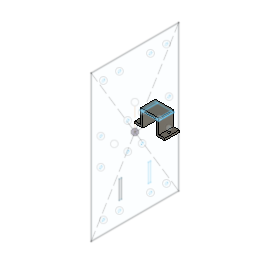
Chassis frame v6-2 (Autodesk Fusion 360 design; units mm, degrees)
Autodesk Fusion 360 part; units mm, degrees
sketch "Sketch1" plane through (0, 0, 0) normal (1, 0, 0) x (0, 1, 0) in component "Integrated frame"
  circle A0 centre (-46.8244, 18.5) radius 1.5
  circle A1 centre (-9.8244, 18.5) radius 1.5
  circle A2 centre (-46.8244, -18.5) radius 1.5
  circle A3 centre (-9.8244, -18.5) radius 1.5
  line L0 (0, 0) -> (0, 35.4619) construction
  line L1 (60, 100) -> (-60, 100)
  line L2 (-60, 100) -> (-60, -100)
  line L3 (-60, -100) -> (60, -100)
  line L4 (60, -100) -> (60, 100)
  line L5 (60, 100) -> (-60, -100) construction
  line L6 (-60, 100) -> (60, -100) construction
  circle A4 centre (46.8244, 18.5) radius 1.5
  circle A5 centre (46.8244, -18.5) radius 1.5
  circle A6 centre (9.8244, -18.5) radius 1.5
  circle A7 centre (9.8244, 18.5) radius 1.5
  line L7 (-18.5, -45.3481) -> (-21.5, -45.3481)
  line L8 (-21.5, -45.3481) -> (-21.5, -70.3481)
  line L9 (-21.5, -70.3481) -> (-18.5, -70.3481)
  line L10 (-18.5, -70.3481) -> (-18.5, -45.3481)
  line L11 (21.5, -45.3481) -> (21.5, -70.3481)
  line L12 (18.5, -70.3481) -> (18.5, -45.3481)
  line L13 (18.5, -45.3481) -> (21.5, -45.3481)
  line L14 (21.5, -70.3481) -> (18.5, -70.3481)
  circle A8 centre (-43.3091, 82.7998) radius 1.5
  circle A9 centre (-21.3091, 82.7998) radius 1.5
  circle A10 centre (21.3091, 82.7998) radius 1.5
  circle A11 centre (43.3091, 82.7998) radius 1.5
  line L15 (0, 0) -> (33.4715, 0) construction
  circle A12 centre (-43.3091, -82.7998) radius 1.5
  circle A13 centre (-21.3091, -82.7998) radius 1.5
  circle A14 centre (43.3091, -82.7998) radius 1.5
  circle A15 centre (21.3091, -82.7998) radius 1.5
  point P0 (-28.3244, 0)
  dimension "d246" = 3
  dimension "d248" = 18.5
  dimension "d249" = 18.5
  dimension "d252" = 37
  dimension "d253" = -37
  dimension "d261" = 120
  dimension "d262" = 200
  dimension "d264" = 3
  dimension "d265" = 25
  dimension "d266" = 18.5
  dimension "d269" = 3
  dimension "d270" = 3
  dimension "d271" = 22
  constraint coincident L0.start L15.start
  constraint horizontal L1
  constraint perpendicular L1 L2
  constraint parallel L1 L3
  constraint parallel L2 L4
  constraint coincident L5 L0.start
  constraint coincident L6 L0.start
  constraint symmetric A0 L0 A4
  constraint symmetric A1 L0 A7
  constraint symmetric A2 L0 A5
  constraint symmetric A3 L0 A6
  constraint horizontal P0 L0.start
  constraint horizontal L7
  constraint vertical L8
  constraint horizontal L9
  constraint vertical L10
  constraint symmetric L0 L7.start L12.end
  constraint symmetric L0 L7.end L11.start
  constraint symmetric L0 L8.end L11.end
  constraint symmetric L0 L9.end L12.start
  constraint horizontal A8.centre A9.centre
  constraint symmetric L0 A8 A11
  constraint symmetric L0 A9 A10
  constraint perpendicular L4 L15
  constraint symmetric A8 L15 A12
  constraint symmetric A9 L15 A13
  constraint symmetric L0 A12 A14
  constraint symmetric L0 A13 A15
  measures "d246" diameter of A0
  measures "d248" horizontal distance of A0.centre P0
  measures "d249" vertical distance of A0.centre P0
  measures "d261" distance of L2.end L3.end
  measures "d262" distance of L1.end L2.end
  measures "d264" distance of L7.start L7.end
  measures "d265" distance of L7.start L9.end
  measures "d266" distance of L0.start L10
  measures "d269" diameter of A8
  measures "d270" diameter of A9
  measures "d271" horizontal distance of A8.centre A9.centre
sketch "Sketch1 (2)" plane through (0, 0, 0) normal (0, 0, 1) x (1, 0, 0) in component "MotorClamp"
  line L0 (0, 50) -> (-19, 50)
  line L1 (-19, 50) -> (-19, 30)
  line L2 (-19, 30) -> (0, 30)
  line L3 (0, 30) -> (0, 50)
  line L4 (-19, 50) -> (-22, 50)
  line L5 (-22, 50) -> (-22, 30)
  line L6 (-22, 30) -> (-19, 30)
  line L7 (-19, 30) -> (-19, 50)
  line L8 (0, 50) -> (3, 50)
  line L9 (3, 50) -> (3, 30)
  line L10 (3, 30) -> (0, 30)
  line L11 (0, 30) -> (0, 50)
  dimension "d272" = 19
  dimension "d273" = 20
  dimension "d274" = 3
  dimension "d275" = 3
  constraint horizontal L0
  constraint vertical L1
  constraint horizontal L2
  constraint vertical L3
  constraint horizontal L4
  constraint vertical L5
  constraint horizontal L6
  constraint vertical L7
  constraint horizontal L8
  constraint vertical L9
  constraint horizontal L10
  constraint vertical L11
  measures "d272" distance of L0.start L0.end
  measures "d273" distance of L0.start L2.end
  measures "d274" distance of L0.end L4.end
  measures "d275" distance of L0.start L8.end
extrude "Extrude1" add sketch "Sketch1 (2)" along normal blind 3 in component "MotorClamp"
extrude "Extrude2" add sketch "Sketch1 (2)" against normal blind 17 contours L3 L8 L9 L10 L11 | L1 L4 L5 L6 L7 in component "MotorClamp"
extrude "Extrude3" add 2 faces at (-20, 36.6667, -17) (1, 43.3333, -17) along direction (0, 0, -1) blind 3 in component "MotorClamp"
sketch "Sketch2" plane through (0, 0, -20) normal (0, 0, -1) x (1, 0, 0) in component "MotorClamp"
  line L0 (-19, -50) -> (-19, -30)
  line L1 (-19, -30) -> (-22, -30)
  line L2 (-22, -30) -> (-22, -50)
  line L3 (-22, -50) -> (-19, -50)
  line L4 (-22, -30) -> (-30, -30)
  line L5 (-30, -30) -> (-30, -50)
  line L6 (-30, -50) -> (-22, -50)
  line L7 (-22, -50) -> (-22, -30)
  line L8 (3, -50) -> (11, -50)
  line L9 (11, -50) -> (11, -30)
  line L10 (11, -30) -> (3, -30)
  line L11 (3, -30) -> (3, -50)
  line L12 (-30, -30) -> (-22, -50) construction
  line L13 (-30, -50) -> (-22, -30) construction
  line L14 (3, -30) -> (11, -50) construction
  line L15 (3, -50) -> (11, -30) construction
  circle A0 centre (-26, -40) radius 1.55
  circle A1 centre (7, -40) radius 1.55
  dimension "d282" = 8
  dimension "d283" = 8
  dimension "d284" = 25
  dimension "d285" = 3.1
  dimension "d286" = 3.1
  constraint horizontal L4
  constraint vertical L5
  constraint horizontal L6
  constraint vertical L7
  constraint coincident L1.end L2.start
  constraint horizontal L8
  constraint vertical L9
  constraint horizontal L10
  constraint vertical L11
  constraint midpoint L12 A0.centre
  constraint midpoint L14 A1.centre
  measures "d282" distance of L1.end L4.end
  measures "d283" distance of L8.start L8.end
  measures "d284" distance of L7 L11
  measures "d285" diameter of A0
  measures "d286" diameter of A1
extrude "Extrude4" add sketch "Sketch2" against normal blind 3 contours L2 L4 L5 L6 L7 | L8 L9 L10 L11 in component "MotorClamp"
extrude "Extrude1'" [suppressed] in component "Integrated frame"
sketch "Laser cut sketch" plane through (3, 0, 0) normal (1, 0, 0) x (0, 1, 0) in component "Integrated frame"
  circle A0 centre (-9.8244, -18.5) radius 1.5
  circle A1 centre (-46.8244, -18.5) radius 1.5
  circle A2 centre (-46.8244, 18.5) radius 1.5
  circle A3 centre (-9.8244, 18.5) radius 1.5
  circle A4 centre (46.8244, 18.5) radius 1.5
  circle A5 centre (46.8244, -18.5) radius 1.5
  circle A6 centre (9.8244, -18.5) radius 1.5
  circle A7 centre (9.8244, 18.5) radius 1.5
  line L0 (-18.5, -45.3481) -> (-18.5, -70.3481)
  line L1 (-18.5, -70.3481) -> (-21.5, -70.3481)
  line L2 (-21.5, -70.3481) -> (-21.5, -45.3481)
  line L3 (-21.5, -45.3481) -> (-18.5, -45.3481)
  line L4 (21.5, -45.3481) -> (21.5, -70.3481)
  line L5 (21.5, -70.3481) -> (18.5, -70.3481)
  line L6 (18.5, -70.3481) -> (18.5, -45.3481)
  line L7 (18.5, -45.3481) -> (21.5, -45.3481)
  line L8 (60, -100) -> (60, 100)
  line L9 (60, 100) -> (-60, 100)
  line L10 (-60, 100) -> (-60, -100)
  line L11 (-60, -100) -> (60, -100)
extrude "Extrude2'" [suppressed]
component "Integrated frame" placed x (1, 0, 0) y (0, 1, 0) z (0, 0, 1) at (0, 0, 0)
component "MotorClamp" placed x (1, 0, 0) y (0, 1, 0) z (0, 0, 1) at (0, 0, 0)
equation "partLength = 250 mm"
equation "partWidth = 25 mm"
equation "boltHole = 3 mm"
equation "boltFromEdgesClose = 10 mm"
equation "boltGap = 12 mm"
equation "boltFromEdgesFar = 40 mm"
equation "boltGapFromSide = ( partWidth - boltGap ) / 2"
equation "boltGapDiag = boltGap * sqrt(2)"
equation "d246 = boltHole"
equation "d248 = ( 37 / 2 ) * 1 mm"
equation "d249 = ( 37 / 2 ) * 1 mm"
equation "d266 = ( 37 / 2 ) * 1 mm"
equation "d269 = boltHole"
equation "d270 = boltHole"
equation "d285 = boltHole + 0.1 mm"
equation "d286 = boltHole + 0.1 mm"
